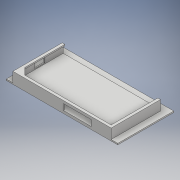
# Autodesk Inventor part: phoneHolder
Saved by Autodesk Inventor 2018 (Build 220112000, 112)
## iProperties
Created: 2017-12-27
Part Number: phoneHolder
Material: Generic
Document SubType Name: Modeling
Designer: mzhang
Density: 1 g/cm^3
Appearance: Default
Author: mzhang
Autodesk Inventor part; units mm, degrees
ref_plane "YZ Plane" through (0, 0, 0) normal (1, 0, 0) x (0, 1, 0)
ref_plane "XZ Plane" through (0, 0, 0) normal (0, 1, 0) x (-1, 0, 0)
ref_plane "XY Plane" through (0, 0, 0) normal (0, 0, 1) x (1, 0, 0)
sketch "Sketch1" plane through (0, 0, 0) normal (0, 0, 1) x (1, 0, 0)
  line L0 (0, 0) -> (144.4, 0)
  line L1 (144.4, 0) -> (144.4, 72)
  line L2 (144.4, 72) -> (0, 72)
  line L3 (0, 72) -> (0, 0)
  line L4 (-0.5, 72.5) -> (144.9, 72.5)
  line L5 (144.9, 72.5) -> (144.9, -0.5)
  line L6 (144.9, -0.5) -> (-0.5, -0.5)
  line L7 (-0.5, -0.5) -> (-0.5, 72.5)
  line L8 (146.4, 72.5) -> (146.4, -2)
  line L9 (146.4, -2) -> (-2, -2)
  line L10 (-2, -2) -> (-2, 72.5)
  line L11 (-2, 72.5) -> (146.4, 72.5)
  dimension "d0" = 144.4
  dimension "d1" = 72
  dimension "d2" = 0.5
  dimension "d3" = 1.5
  constraints: 24 end point, 5 parallel, 3 perpendicular, 1 horizontal, 1 point on line, 3 other
  measures "d0" distance of L2.end L1.end
  measures "d1" distance of L1.end L0.end
  measures "d2" distance between parallel lines of L2 L4
  measures "d3" distance between parallel lines of L7 L10
extrude "Extrusion1" add sketch "Sketch1" along normal blind 11 contours L7 L6 L5 L11 L8 L9 L10
sketch "Sketch2" plane through (0, 0, 11) normal (0, 0, 1) x (1, 0, 0)
  line L0 (-2, 72.5) -> (-2, -2) projected
  line L1 (-2, 72.5) -> (-2, -2)
  line L2 (-2, -2) -> (146.4, -2) projected
  line L3 (-2, -2) -> (146.4, -2)
  line L4 (146.4, -2) -> (146.4, 72.5) projected
  line L5 (146.4, -2) -> (146.4, 72.5)
  line L6 (-2, 72.5) -> (2, 72.5)
  line L7 (2, 72.5) -> (2, 2)
  line L8 (-0.5, -0.5) -> (-0.5, 72.5) projected
  line L9 (146.4, 72.5) -> (142.4, 72.5)
  line L10 (2, 2) -> (142.4, 2)
  line L11 (142.4, 72.5) -> (142.4, 2)
  point P0 (0, 0)
  dimension "d6" = 4
  dimension "d7" = 4
  constraints: 16 end point, 3 perpendicular, 2 collinear, 1 horizontal, 1 parallel, 1 vertical
  measures "d6" distance of L0.start L6.end
  measures "d7" distance of L4.end L9.end
extrude "Extrusion2" add sketch "Sketch2" along normal blind 2
sketch "Sketch3" plane through (0, 0, 0) normal (0, 0, -1) x (-1, 0, 0)
  line L0 (-146.4, -2) -> (-146.4, 72.5) projected
  line L1 (2, 72.5) -> (2, -2) projected
  line L2 (-146.4, 72.5) -> (2, 72.5)
  line L3 (2, 72.5) -> (2, -2)
  line L4 (2, -2) -> (-146.4, -2)
  line L5 (-146.4, -2) -> (-146.4, 72.5)
  point P0 (0, 0)
  constraints: 8 end point, 2 parallel, 1 horizontal, 1 perpendicular
extrude "Extrusion3" add sketch "Sketch3" along normal blind 2
sketch "Sketch4" plane through (0, 0, -2) normal (0, 0, -1) x (-1, 0, 0)
  line L0 (2, 72.5) -> (-146.4, 72.5) projected
  line L1 (-146.4, 72.5) -> (-146.4, -2) projected
  line L2 (-146.4, -2) -> (2, -2) projected
  line L3 (2, -2) -> (2, 72.5) projected
  line L4 (-156.4, 82.5) -> (12, 82.5)
  line L5 (12, 82.5) -> (12, -2)
  line L6 (-156.4, -2) -> (-156.4, 82.5)
  line L7 (-146.4, -2) -> (2, -2) projected
  line L8 (-146.4, -2) -> (-156.4, -2)
  line L9 (2, -2) -> (2, 72.5) projected
  line L10 (2, -2) -> (12, -2)
  point P0 (0, 0)
  dimension "d12" = 10
  constraints: 10 end point, 2 point on line
  measures "d12" distance between parallel lines of L0 L4
extrude "Extrusion4" add sketch "Sketch4" along normal blind 2
sketch "Sketch5" plane through (-2, -2, 13) normal (-1, 0, 0) x (0, 0, 1)
  line L0 (0, 74.5) -> (0, 4) projected
  line L1 (0, 74.5) -> (-15, 74.5) projected
  line L2 (-3.5, 31.75) -> (-11.5, 31.75)
  line L3 (-11.5, 31.75) -> (-11.5, 46.75)
  line L4 (-11.5, 46.75) -> (-3.5, 46.75)
  line L5 (-3.5, 46.75) -> (-3.5, 31.75)
  line L6 (-3.5, 31.75) -> (-11.5, 46.75) construction
  line L7 (-11.5, 31.75) -> (-3.5, 46.75) construction
  point P0 (-13, 2)
  point P1 (0, 39.25)
  point P2 (-7.5, 74.5)
  point P3 (-7.5, 39.25)
  dimension "d15" = 8
  dimension "d16" = 15
  constraints: 12 end point, 4 midpoint, 2 parallel, 1 horizontal, 1 perpendicular
  measures "d15" distance of L3.end L4.end
  measures "d16" distance of L2.end L3.end
extrude "Extrusion5" cut sketch "Sketch5" against normal up to surface (1.5 mm away)
sketch "Sketch6" plane through (-0.5, -0.5, 11) normal (0, 1, 0) x (1, 0, 0)
  line L0 (0, 11) -> (145.4, 11) projected
  line L1 (116.9, 2) -> (74.9, 2)
  line L2 (74.9, 2) -> (74.9, 11)
  line L3 (74.9, 11) -> (116.9, 11)
  line L4 (116.9, 11) -> (116.9, 2)
  point P0 (0.5, 11)
  dimension "d19" = 42
  constraints: 8 end point, 2 parallel, 1 horizontal, 1 perpendicular, 1 point on line
  measures "d19" distance of L2.end L3.end
extrude "Extrusion6" cut sketch "Sketch6" against normal up to surface (1.5 mm away)
chamfer "Chamfer1" distance 10 angle 45 1 edges at (2, 2, 12)
body "Solid1"
